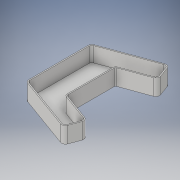
# Autodesk Inventor part: CONTROLLER CASE
Saved by Autodesk Inventor 2019.4 (Build 234330000, 330)
## iProperties
Created: 2019-06-21
Part Number: CONTROLLER CASE
Material: Generic
Document SubType Name: Modeling
Designer: abdel
Density: 1 g/cm^3
Appearance: Default
Author: abdel
Autodesk Inventor part; units mm, degrees
ref_plane "YZ Plane" through (0, 0, 0) normal (1, 0, 0) x (0, 1, 0)
ref_plane "XZ Plane" through (0, 0, 0) normal (0, 1, 0) x (-1, 0, 0)
ref_plane "XY Plane" through (0, 0, 0) normal (0, 0, 1) x (1, 0, 0)
sketch "Sketch1" plane through (0, 0, 0) normal (0, 1, 0) x (-1, 0, 0)
  circle A0 centre (34.925, 5.5508) radius 13.97
  line L0 (69.85, 28.9263) -> (69.85, -106.7248)
  line L1 (0, -91.6029) -> (0, 13.8044)
  line L2 (-4.1782, 19.7715) -> (-65.6375, 42.1409)
  line L3 (-4.1782, -97.57) -> (-65.6375, -119.9394)
  line L4 (65.6718, 34.8933) -> (-52.6066, 77.9431)
  line L5 (65.6718, -112.6918) -> (-52.6066, -155.7416)
  line L6 (-69.4327, 50.2797) -> (-60.7454, 74.1479)
  line L7 (-69.4327, -128.0782) -> (-60.7454, -151.9464)
  arc A1 (-69.4327, 50.2797) -> (-65.6375, 42.1409) centre (-63.4657, 48.1079) ccw
  arc A2 (-52.6066, 77.9431) -> (-60.7454, 74.1479) centre (-54.7784, 71.9761) ccw
  arc A3 (-65.6375, -119.9394) -> (-69.4327, -128.0782) centre (-63.4657, -125.9064) ccw
  arc A4 (-60.7454, -151.9464) -> (-52.6066, -155.7416) centre (-54.7784, -149.7746) ccw
  arc A5 (69.85, 28.9263) -> (65.6718, 34.8933) centre (63.5, 28.9263) ccw
  arc A6 (65.6718, -112.6918) -> (69.85, -106.7248) centre (63.5, -106.7248) ccw
  arc A7 (-4.1782, -97.57) -> (0, -91.6029) centre (-6.35, -91.6029) ccw
  arc A8 (0, 13.8044) -> (-4.1782, 19.7715) centre (-6.35, 13.8044) ccw
  line L8 (-51.7378, 80.33) -> (66.5406, 37.2802)
  arc A9 (72.39, 28.9263) -> (66.5406, 37.2802) centre (63.5, 28.9263) ccw
  line L9 (72.39, 28.9263) -> (72.39, -106.7248)
  arc A10 (66.5406, -115.0786) -> (72.39, -106.7248) centre (63.5, -106.7248) ccw
  line L10 (66.5406, -115.0786) -> (-51.7378, -158.1285)
  arc A11 (-63.1323, -152.8152) -> (-51.7378, -158.1285) centre (-54.7784, -149.7746) ccw
  line L11 (-63.1323, -152.8152) -> (-71.8196, -128.947)
  arc A12 (-66.5063, -117.5525) -> (-71.8196, -128.947) centre (-63.4657, -125.9064) ccw
  line L12 (-66.5063, -117.5525) -> (-5.0469, -95.1832)
  arc A13 (-5.0469, -95.1832) -> (-2.54, -91.6029) centre (-6.35, -91.6029) ccw
  line L13 (-2.54, -91.6029) -> (-2.54, 13.8044)
  arc A14 (-2.54, 13.8044) -> (-5.0469, 17.3847) centre (-6.35, 13.8044) ccw
  line L14 (-5.0469, 17.3847) -> (-66.5063, 39.754)
  arc A15 (-71.8196, 51.1485) -> (-66.5063, 39.754) centre (-63.4657, 48.1079) ccw
  line L15 (-71.8196, 51.1485) -> (-63.1323, 75.0167)
  arc A16 (-51.7378, 80.33) -> (-63.1323, 75.0167) centre (-54.7784, 71.9761) ccw
  point P0 (0, 0)
  point P1 (0, 0)
  point P2 (0, 18.2508)
  point P3 (0, -96.0492)
  point P4 (-71.6046, 44.3127)
  point P5 (-71.6046, -122.1112)
  point P6 (69.85, 33.3726)
  point P7 (-58.5736, 80.115)
  point P8 (69.85, -111.1711)
  point P9 (-58.5736, -157.9135)
  dimension "d0" = 27.94
  dimension "d1" = 114.3
  dimension "d2" = 76.2
  dimension "d3" = 110
  dimension "d4" = 76.2
  dimension "d5" = 110
  dimension "d6" = 38.1
  dimension "d7" = 38.1
  dimension "d8" = 34.925
  dimension "d9" = 12.7
  dimension "d10" = 6.35
  dimension "d11" = 6.35
  dimension "d12" = 69.85
  dimension "d13" = 2.54
  constraints: 32 end point, 32 point on circle, 17 centre point, 16 point on line, 16 tangent, 6 equal radius, 6 parallel, 15 other
  measures "d0" diameter of A0
  measures "d1" distance of point (0, -96.049) point (0, 18.251)
  measures "d2" distance of point (0, 18.251) point (-71.605, 44.313)
  measures "d3" angle of L2 L1
  measures "d4" distance of point (0, -96.049) point (-71.605, -122.111)
  measures "d5" angle of L3 L1
  measures "d6" distance between parallel lines of L2 L4
  measures "d7" distance between parallel lines of L3 L5
  measures "d8" distance from line of L1 A0.centre
  measures "d9" vertical distance of point (0, 18.251) A0.centre
  measures "d10" radius of A1
  measures "d11" radius of A5
  measures "d12" distance between parallel lines of L0 L1
  measures "d13" distance between parallel lines of L4 L8
extrude "Extrusion1" add sketch "Sketch1" along normal blind 36.83 contours L8 A9 L9 A10 L10 A11 L11 A12 L12 A13 L13 A14 L14 A15 L15 A16
sketch "Sketch4" plane through (0, 0, 0) normal (0, 1, 0) x (-1, 0, 0)
  arc A0 (65.6718, -112.6918) -> (69.85, -106.7248) centre (63.5, -106.7248) ccw
  line L0 (-4.1782, -97.57) -> (-65.6375, -119.9394)
  line L1 (65.6718, -112.6918) -> (-52.6066, -155.7416)
  arc A1 (-4.1782, -97.57) -> (0, -91.6029) centre (-6.35, -91.6029) ccw
  line L2 (-4.1782, 19.7715) -> (-65.6375, 42.1409)
  arc A2 (-65.6375, -119.9394) -> (-69.4327, -128.0782) centre (-63.4657, -125.9064) ccw
  line L3 (-69.4327, -128.0782) -> (-60.7454, -151.9464)
  arc A3 (-60.7454, -151.9464) -> (-52.6066, -155.7416) centre (-54.7784, -149.7746) ccw
  line L4 (0, -91.6029) -> (0, 13.8044)
  line L5 (69.85, 28.9263) -> (69.85, -106.7248)
  arc A4 (0, 13.8044) -> (-4.1782, 19.7715) centre (-6.35, 13.8044) ccw
  arc A5 (69.85, 28.9263) -> (65.6718, 34.8933) centre (63.5, 28.9263) ccw
  line L6 (65.6718, 34.8933) -> (-52.6066, 77.9431)
  line L7 (-69.4327, 50.2797) -> (-60.7454, 74.1479)
  arc A6 (-52.6066, 77.9431) -> (-60.7454, 74.1479) centre (-54.7784, 71.9761) ccw
  arc A7 (-69.4327, 50.2797) -> (-65.6375, 42.1409) centre (-63.4657, 48.1079) ccw
  line L8 (-51.7378, 80.33) -> (66.5406, 37.2802)
  arc A8 (72.39, 28.9263) -> (66.5406, 37.2802) centre (63.5, 28.9263) ccw
  line L9 (72.39, 28.9263) -> (72.39, -106.7248)
  arc A9 (66.5406, -115.0786) -> (72.39, -106.7248) centre (63.5, -106.7248) ccw
  line L10 (66.5406, -115.0786) -> (-51.7378, -158.1285)
  arc A10 (-63.1323, -152.8152) -> (-51.7378, -158.1285) centre (-54.7784, -149.7746) ccw
  line L11 (-63.1323, -152.8152) -> (-71.8196, -128.947)
  arc A11 (-66.5063, -117.5525) -> (-71.8196, -128.947) centre (-63.4657, -125.9064) ccw
  line L12 (-66.5063, -117.5525) -> (-5.0469, -95.1832)
  arc A12 (-5.0469, -95.1832) -> (-2.54, -91.6029) centre (-6.35, -91.6029) ccw
  line L13 (-2.54, -91.6029) -> (-2.54, 13.8044)
  arc A13 (-2.54, 13.8044) -> (-5.0469, 17.3847) centre (-6.35, 13.8044) ccw
  line L14 (-5.0469, 17.3847) -> (-66.5063, 39.754)
  arc A14 (-71.8196, 51.1485) -> (-66.5063, 39.754) centre (-63.4657, 48.1079) ccw
  line L15 (-71.8196, 51.1485) -> (-63.1323, 75.0167)
  arc A15 (-51.7378, 80.33) -> (-63.1323, 75.0167) centre (-54.7784, 71.9761) ccw
  point P0 (0, 0)
  point P1 (0, 0)
  point P2 (0, -96.0492)
  point P3 (69.85, -111.1711)
  point P4 (-71.6046, -122.1112)
  point P5 (-58.5736, -157.9135)
  point P6 (0, 18.2508)
  point P7 (-71.6046, 44.3127)
  point P8 (69.85, 33.3726)
  point P9 (-58.5736, 80.115)
  point P10 (0, 0)
  dimension "d17" = 114.3
  dimension "d18" = 76.2
  dimension "d19" = 110
  dimension "d20" = 76.2
  dimension "d21" = 110
  dimension "d22" = 38.1
  dimension "d23" = 38.1
  dimension "d26" = 6.35
  dimension "d27" = 6.35
  dimension "d28" = 69.85
  dimension "d29" = 2.54
  constraints: 32 end point, 32 point on circle, 16 centre point, 16 point on line, 16 tangent, 6 equal radius, 6 parallel, 15 other
  measures "d17" distance of point (0, -96.049) point (0, 18.251)
  measures "d18" distance of point (0, 18.251) point (-71.605, 44.313)
  measures "d19" angle of L2 L4
  measures "d20" distance of point (0, -96.049) point (-71.605, -122.111)
  measures "d21" angle of L0 L4
  measures "d22" distance between parallel lines of L2 L6
  measures "d23" distance between parallel lines of L0 L1
  measures "d26" radius of A7
  measures "d27" radius of A5
  measures "d28" distance between parallel lines of L5 L4
  measures "d29" distance between parallel lines of L6 L8
extrude "Extrusion2" add sketch "Sketch4" along normal blind 2.54 contours L1 A3 L3 A2 L0 A1 L4 A4 L2 A7 L7 A6 L6 A5 L5 A0
body "Solid1"
